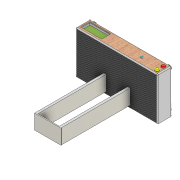
# Autodesk Inventor part: base 2
Saved by Autodesk Inventor 2021 (Build 250183000, 183)
## iProperties
Created: 2021-06-25
Part Number: base 2
Material: Generic
Document SubType Name: Modeling
Designer: Nikita
Density: 1 g/cm^3
Appearance: Engine Turned
Author: Nikita
Autodesk Inventor part; units mm, degrees
ref_plane "YZ Plane" through (0, 0, 0) normal (1, 0, 0) x (0, 1, 0)
ref_plane "XZ Plane" through (0, 0, 0) normal (0, 1, 0) x (-1, 0, 0)
ref_plane "XY Plane" through (0, 0, 0) normal (0, 0, 1) x (1, 0, 0)
sketch "Sketch1" plane through (0, 0, 0) normal (0, 0, 1) x (1, 0, 0)
  line L0 (-14.39, 90) -> (155.61, 90)
  line L1 (155.61, 90) -> (155.61, 0)
  line L2 (155.61, 0) -> (-14.39, 0)
  line L3 (-14.39, 0) -> (-14.39, 90)
  point P0 (0, 0)
  dimension "d0" = 170
  dimension "d1" = 90
  constraints: 8 end point, 2 parallel, 1 horizontal, 1 perpendicular
  measures "d0" distance of L1.end L2.end
  measures "d1" distance of L2.end L0.start
extrude "Extrusion1" add sketch "Sketch1" along normal blind 30
fillet "Fillet1" radius 2 11 edges at (70.61, 90, 0) (155.61, 90, 15) (70.61, 90, 30) (155.61, 45, 0) (155.61, 45, 30) (70.61, 0, 0) (70.61, 0, 30) (-14.39, 0, 15) (-14.39, 45, 30) (-14.39, 45, 0) (-14.39, 90, 15)
sketch "Sketch2" plane through (-12.39, 90, 2) normal (0, 1, 0) x (1, 0, 0)
  circle A0 centre (160.2339, -7.6328) radius 4
  circle A1 centre (160.2339, -20.316) radius 4
  point P0 (12.39, 2)
  constraints: 2 centre point
extrude "Extrusion2" add sketch "Sketch2" along normal blind 2.5
fillet "Fillet2" radius 1.5 2 edges at (143.844, 92.5, 22.316) (143.844, 92.5, 9.6328)
sketch "Sketch3" plane through (0, 0, 0) normal (0, 0, -1) x (-1, 0, 0)
  line L0 (-155.61, 0) -> (-147.61, 0)
  line L1 (12.39, 0) -> (-155.61, 0) projected
  circle A0 centre (-147.61, 82.5757) radius 4.25
  circle A1 centre (-147.61, 8) radius 4.25
  circle A2 centre (7.5895, 8) radius 4.25
  circle A3 centre (7.5895, 82.5757) radius 4.25
  point P0 (0, 0)
  constraints: 4 centre point, 2 end point, 1 point on line
extrude "Extrusion3" add sketch "Sketch3" along normal blind 4
fillet "Fillet3" radius 1 4 edges at (151.86, 82.5757, -4) (151.86, 8, -4) (-3.3395, 8, -4) (-3.3395, 82.5757, -4)
sketch "Sketch4" plane through (-12.39, 90, 2) normal (0, 1, 0) x (1, 0, 0)
  line L0 (46.649, -22.3484) -> (2.8464, -22.3484)
  line L1 (2.8464, -22.3484) -> (2.8464, -3.0165)
  line L2 (2.8464, -3.0165) -> (46.649, -3.0165)
  line L3 (46.649, -3.0165) -> (46.649, -22.3484)
  point P0 (12.39, 2)
  constraints: 8 end point, 2 parallel, 1 horizontal, 1 perpendicular
extrude "Extrusion4" cut sketch "Sketch4" against normal blind 4
chamfer "Chamfer1" distance 2 angle 45 4 edges at (34.259, 86, 14.6824) (12.3577, 86, 5.0165) (-9.5436, 86, 14.6824) (12.3577, 86, 24.3484)
sketch "Sketch5" plane through (-14.39, 2, 2) normal (-1, 0, 0) x (0, 0, 1)
  point P0 (-2, -2)
sketch "Sketch6" plane through (0, 0, 30) normal (0, 0, 1) x (1, 0, 0)
  line L0 (-14.39, 88) -> (-14.39, 2) projected
  line L1 (44.515, 37.023) -> (49.3226, 37.023)
  line L2 (49.3226, 37.023) -> (49.3226, 6.119)
  line L3 (49.3226, 6.119) -> (44.515, 6.119)
  line L4 (44.515, 6.119) -> (44.515, 37.023)
  line L5 (155.61, 0) -> (155.61, 88) projected
  line L6 (98.364, 37.023) -> (93.364, 37.023)
  line L7 (93.364, 37.023) -> (93.364, 6.119)
  line L8 (93.364, 6.119) -> (98.364, 6.119)
  line L9 (98.364, 6.119) -> (98.364, 37.023)
  point P0 (0, 0)
  constraints: 16 end point, 4 parallel, 2 horizontal, 2 perpendicular
extrude "Extrusion5" add sketch "Sketch6" along normal blind 144 contours L1 L2 L3 L4
sketch "Sketch7" plane through (0, 0, 30) normal (0, 0, 1) x (1, 0, 0)
  line L0 (44.515, 37.023) -> (49.3226, 37.023) projected
  line L1 (49.3226, 6.119) -> (44.515, 6.119) projected
  line L2 (98.8996, 37.023) -> (93.8996, 37.023)
  line L3 (93.8996, 37.023) -> (93.8996, 6.119)
  line L4 (93.8996, 6.119) -> (98.8996, 6.119)
  line L5 (98.8996, 6.119) -> (98.8996, 37.023)
  point P0 (0, 0)
  constraints: 8 end point, 2 parallel, 1 horizontal, 1 perpendicular
extrude "Extrusion6" add sketch "Sketch7" along normal blind 142
sketch "Sketch8" plane through (49.3226, 6.119, 30) normal (1, 0, 0) x (0, 0, -1)
  line L0 (0, 30.904) -> (-144, 30.904) projected
  line L1 (-142, 30.904) -> (-142, 0) projected
  line L2 (-144, 30.904) -> (-142, 30.904)
  line L3 (-142, 30.904) -> (-142, 0)
  line L4 (-142, 0) -> (-144, 0)
  line L5 (-144, 0) -> (-144, 30.904)
  point P0 (30, -6.119)
  constraints: 8 end point, 2 parallel, 1 horizontal, 1 perpendicular
extrude "Extrusion7" add sketch "Sketch8" along normal blind 50
sketch "Sketch9" plane through (-12.39, 90, 2) normal (0, 1, 0) x (1, 0, 0)
  circle A0 centre (121.1087, -13.5546) radius 2
  point P0 (12.39, 2)
  constraints: 1 centre point
extrude "Extrusion8" add sketch "Sketch9" along normal blind 4
fillet "Fillet4" radius 2 1 edges at (106.7188, 94, 15.5546)
body "Solid1"
